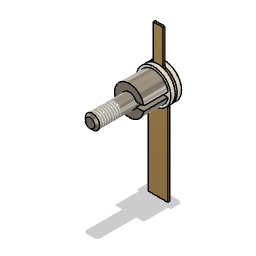
pulse transfer v23 (Autodesk Fusion 360 design; units mm, degrees)
Autodesk Fusion 360 part; units mm, degrees
sketch "Sketch1" plane through (0, 0, 0) normal (0, 1, 0) x (1, 0, 0)
  line L0 (1.5, 13) -> (3, 13)
  line L1 (3, 13) -> (3, 8)
  line L2 (3, 8) -> (1.5, 8)
  line L3 (1.5, 8) -> (1.5, 0)
  line L4 (1.5, 0) -> (0, 0)
  line L5 (0, 0) -> (0, 15.5)
  line L6 (0, 15.5) -> (3, 15.5)
  line L7 (1.5, 8) -> (1.5, 13)
  line L8 (3, 15.5) -> (3, 15)
  line L9 (3, 15) -> (1.5, 15)
  line L10 (1.5, 15) -> (1.5, 13)
  dimension "d1" = 3
  dimension "d2" = 1.5
  dimension "d3" = 8
  dimension "d4" = 5
  dimension "d26" = 0.5
  dimension "d27" = 2
  constraint perpendicular L0 L1
  constraint perpendicular L2 L3
  constraint perpendicular L4 L5
  constraint coincident L4.end L5.start
  constraint vertical L5
  constraint vertical L7
  constraint horizontal L6
  constraint perpendicular L6 L8
  constraint perpendicular L7 L9
  constraint perpendicular L0 L10
  constraint collinear L1 L8
  measures "d1" distance of L1 L5
  measures "d2" distance of L3 L5
  measures "d3" distance of L2 L4
  measures "d4" distance of L0 L2
  measures "d26" distance of L6.end L8.end
  measures "d27" distance of L0 L9
revolve "Revolve1" add sketch "Sketch1" angle 360 about axis through (0, 0, 0) along (0, 0, -1) contours L0 L1 L2 L7 makes body 1
revolve "Revolve2" add sketch "Sketch1" angle 360 about axis through (0, 0, 0) along (0, 0, -1) separate body contours L3 L4 L5 L6 L7 L8 L9 L10 makes body 2
sketch "Sketch2" plane through (0, 0, -13) normal (0, 0, -1) x (-1, 0, 0)
  circle A0 centre (0, 0) radius 3
  circle A1 centre (0, 0) radius 3.5
  circle A2 centre (0, 0) radius 1.75
  circle A3 centre (0, 0) radius 1.5
  dimension "d7" = 7
  dimension "d8" = 3.5
  constraint concentric A1 A2
  measures "d7" diameter of A1
  measures "d8" diameter of A2
extrude "Extrude1" add sketch "Sketch2" along normal blind 0.9 separate body contours A0 | A1 makes body 3
sketch "Sketch3" plane through (0, 0, -13.9) normal (0, 0, -1) x (-1, 0, 0)
  circle A0 centre (0, 0) radius 1.75
  circle A1 centre (0, 0) radius 3.5
  line L0 (-3.5, 10.5) -> (3.5, 10.5)
  line L1 (3.5, 10.5) -> (3.5, 0)
  line L2 (-3.5, 0) -> (-3.5, 10.5)
  line L3 (0, 1.75) -> (0, 22.5) construction
  line L4 (-3.5, 3.5) -> (3.5, 3.5) construction
  line L5 (-1, 10.5) -> (-1, 3.3541)
  circle A2 centre (0, 0) radius 3.5
  line L6 (1, 10.5) -> (1, 3.3541)
  circle A3 centre (0, 0) radius 2
  line L7 (2, -2.8723) -> (2, -20)
  line L8 (2, -20) -> (-2, -20)
  line L9 (-2, -20) -> (-2, -2.8723)
  dimension "d14" = 7
  dimension "d15" = 2
  dimension "d34" = 4
  dimension "d36" = 7
  dimension "d37" = 4
  dimension "d38" = 20
  constraint horizontal L0
  constraint perpendicular L0 L1
  constraint perpendicular L0 L2
  constraint symmetric L1 L2 L3
  constraint coincident L2 L4.start
  constraint coincident L1 L4.end
  constraint perpendicular L1 L4
  constraint tangent A1 L4
  constraint coincident L0 L5.start
  constraint perpendicular L0 L5
  constraint coincident L5.end A2
  constraint coincident L0 L6.start
  constraint coincident A2 L6.end
  constraint perpendicular L4 L6
  constraint concentric A2 A3
  constraint coincident L1.end A2
  constraint coincident L2.start A2
  constraint coincident A2 L7.start
  constraint vertical L7
  constraint perpendicular L7 L8
  constraint coincident A2 L9.end
  constraint perpendicular L8 L9
  measures "d14" distance of L0 L4
  measures "d15" distance of L5 L6
  measures "d34" diameter of A3
  measures "d36" distance of L0.start L0.end
  measures "d37" distance of L7.end L8.end
  measures "d38" distance of A0.centre L8
extrude "Extrude2" add sketch "Sketch3" along normal blind 0.38 separate body contours A1 A2 | A1 L0 L5 A2 L6 makes body 4
extrude "Extrude3" add sketch "Sketch3" along normal up to surface (0.38 mm away) contours A1 A2 L7 L8 L9 bodies 4
mirror "Mirror1" about plane through (0, 0, 0) normal (1, 0, 0) of "Extrude3"
fillet "Fillet1" radius 0.4 4 edges at (1, 3.3541, -14.09) (2, -2.8723, -14.09) (-1, 3.3541, -14.09) (-2, -2.8723, -14.09) on bodies 4
thread "Thread2" "ISO Metric profile 3.0 M3x0.5 6g" major diameter 2.927 minor diameter 2.3555 pitch 0.5 angle 60 resizes the face on face at (1.4981, 0.0748, -9.6667) from (0, 0, -5) to (0, 0, 0) on bodies 2
chamfer "Chamfer2" distance 0.5 angle 45 1 edges at (-1.3645, -0.5292, 0) on bodies 2
extrude "Extrude4" cut sketch "Sketch1" along normal mid plane 1 bodies 1
copy_body "Body->Comp1" bodies 1 removing the originals makes body 5 in component "stem"
copy_body "Body->Comp2" bodies 3 removing the originals makes body 6 in component "washer"
copy_body "Body->Comp3" bodies 4 removing the originals makes body 7 in component "conductor"
copy_body "Body->Comp4" bodies 2 removing the originals makes body 8 in component "center pin"
sketch "conductor cutting pattern" plane through (0, 0, -14.28) normal (0, 0, -1) x (-1, 0, 0)
  line L0 (1, 3.6401) -> (1, 10.5)
  line L1 (1, 10.5) -> (-1, 10.5)
  line L2 (-1, 10.5) -> (-1, 3.6401)
  arc A0 (2.1538, -2.7588) -> (1.2564, 3.2667) centre (0, 0) ccw
  arc A1 (-1.2564, 3.2667) -> (-1, 3.6401) centre (-1.4, 3.6401) ccw
  arc A2 (-1.2564, 3.2667) -> (-2.1538, -2.7588) centre (0, 0) ccw
  line L3 (-2, -3.0741) -> (-2, -20)
  line L4 (-2, -20) -> (2, -20)
  line L5 (2, -20) -> (2, -3.0741)
  arc A3 (1, 3.6401) -> (1.2564, 3.2667) centre (1.4, 3.6401) ccw
  arc A4 (-2, -3.0741) -> (-2.1538, -2.7588) centre (-2.4, -3.0741) ccw
  arc A5 (2.1538, -2.7588) -> (2, -3.0741) centre (2.4, -3.0741) ccw
  circle A6 centre (0, 0) radius 2
component "stem" placed x (1, 0, 0) y (0, 1, 0) z (0, 0, 1) at (0, 0, 0)
component "washer" placed x (1, 0, 0) y (0, 1, 0) z (0, 0, 1) at (0, 0, 0)
component "conductor" placed x (1, 0, 0) y (0, 1, 0) z (0, 0, 1) at (0, 0, 0)
component "washer" placed x (1, 0, 0) y (0, 1, 0) z (0, 0, 1) at (0, 0, -1.28)
component "center pin" placed x (1, 0, 0) y (0, 1, 0) z (0, 0, 1) at (0, 0, 0)
named bodies: "stem", "washer", "conductor", "center pin"
